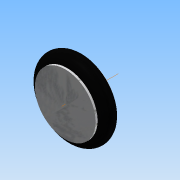
# Autodesk Inventor part: roulement_joint
Saved by Autodesk Inventor 2015 (Build 190159000, 159)
## iProperties
Created: 2016-03-31
Part Number: roulement_joint
Material: Générique
Document SubType Name: Modeling
Designer: Gregwar
Density: 1 g/cm^3
Appearance: Par défaut
Author: Gregwar
Autodesk Inventor part; units mm, degrees
ref_plane "YZ Plane" through (0, 0, 0) normal (1, 0, 0) x (0, 1, 0)
ref_plane "XZ Plane" through (0, 0, 0) normal (0, 1, 0) x (-1, 0, 0)
ref_plane "XY Plane" through (0, 0, 0) normal (0, 0, 1) x (1, 0, 0)
sketch "Esquisse1" plane through (0, 0, 0) normal (0, 1, 0) x (-1, 0, 0)
  circle A0 centre (0, 0) radius 6
  dimension "d0" = 12
  constraints: 1 centre point, 1 coincident
  measures "d0" diameter of A0
extrude "Extrusion1" add sketch "Esquisse1" along normal blind 4
sketch "Esquisse2" plane through (0, 0, 0) normal (1, 0, 0) x (0, 1, 0)
  line L0 (4, -6) -> (4, 6) projected
  line L1 (0, 6) -> (0, -6) projected
  line L2 (0, -6) -> (4, -6) projected
  circle A0 centre (2, -6) radius 1.6
  line L3 (2, -6) -> (2, 10.4927)
  line L4 (2, 0) -> (9.8007, 0)
  line L5 (4, -6) -> (4, 6) projected
  line L6 (4, 0) -> (-2.9892, 0)
  point P0 (0, 0)
  dimension "d3" = 3.2
  constraints: 6 end point, 2 midpoint, 2 point on line, 1 centre point, 1 perpendicular, 1 vertical
  measures "d3" diameter of A0
revolve "Révolution1" add sketch "Esquisse2" angle 360 about axis through (0, 4, 0) along (0, -1, 0) contours A0 L2 | L2 L3 A0 | L2 A0 L3
